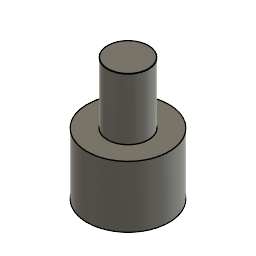
Exercise_4_Problem (Autodesk Fusion 360 design; units mm, degrees)
part number: 2026-05-18-23-14-52-166
Autodesk Fusion 360 part; units mm, degrees
sketch "Sketch1" plane through (0, 0, 0) normal (0, 1, 0) x (1, 0, 0)
  circle A0 centre (0, 0) radius 20
  circle A1 centre (0, 0) radius 10
  dimension "d1" = 40
  dimension "d2" = 20
  constraint coincident A0.centre A1.centre
  constraint concentric A0 A1
  measures "d1" diameter of A0
  measures "d2" diameter of A1
extrude "Extrude1" add sketch "Sketch1" along normal blind 30
extrude "Extrude2" add sketch "Sketch1" along normal blind 60 contours A1
fillet "Fillet1" radius 0.1 1 edges at (-9.3233, 60, 3.6162)
